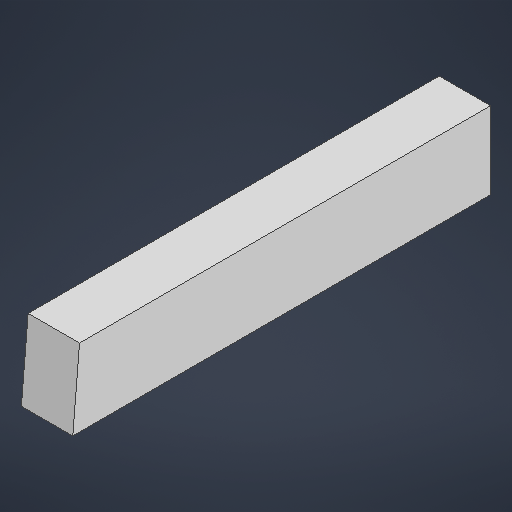
# Autodesk Inventor part: motorstand2
Saved by Autodesk Inventor 2026.2 (Build 302298000, 298)
## iProperties
Created: 2026-02-24
Part Number: motorstand2
Material: Generic
Document SubType Name: Modeling
Designer: danda
Density: 1 g/cm^3
Appearance: Default
Author: danda
Autodesk Inventor part; units mm, degrees
ref_plane "YZ Plane" through (0, 0, 0) normal (1, 0, 0) x (0, 1, 0)
ref_plane "XZ Plane" through (0, 0, 0) normal (0, 1, 0) x (-1, 0, 0)
ref_plane "XY Plane" through (0, 0, 0) normal (0, 0, 1) x (1, 0, 0)
sketch "Sketch1" plane through (0, 0, 0) normal (0, 0, 1) x (1, 0, 0)
  line L0 (22.0768, 43.8051) -> (34.0768, 43.8051)
  line L1 (34.0768, 43.8051) -> (34.0768, 21.8051)
  line L2 (34.0768, 21.8051) -> (22.0768, 21.8051)
  line L3 (22.0768, 21.8051) -> (22.0768, 43.8051)
  line L4 (38.0768, 47.8051) -> (18.0768, 47.8051)
  line L5 (18.0768, 47.8051) -> (18.0768, 17.8051)
  line L6 (18.0768, 17.8051) -> (38.0768, 17.8051)
  line L7 (38.0768, 17.8051) -> (38.0768, 47.8051)
  point P0 (0, 0)
  dimension "d4" = 12
  dimension "d5" = 22
  dimension "d6" = 4
  constraints: 16 end point, 4 parallel, 2 perpendicular, 1 horizontal, 3 other
  measures "d4" distance of L1.end L2.end
  measures "d5" distance of L0.end L1.end
  measures "d6" distance between parallel lines of L0 L4
extrude "Extrusion2" add sketch "Sketch1" along normal blind 100 and the other way blind 60
sketch "Sketch2" plane through (38.0768, 17.8051, 100) normal (1, 0, 0) x (0, 0, -1)
  line L0 (0, 0) -> (0, 30) projected
  line L1 (0, 0) -> (30.1146, 0) construction
  line L2 (0, 30) -> (-2.6247, 0)
  line L3 (0, 30) -> (32.6362, 30) construction
  line L4 (0, 0) -> (-2.6247, 0)
  point P0 (100, -17.8051)
  dimension "d16" = 95
  constraints: 8 end point, 3 horizontal
  measures "d16" angle of L2 L3
extrude "Extrusion3" add sketch "Sketch2" against normal blind 20
body "Solid2"
